J8 (Autodesk Fusion 360 design; units mm, degrees)
part number: 2026-05-31-14-41-56-693
Autodesk Fusion 360 part; units mm, degrees
sketch "Sketch1" plane through (0, 0, 0) normal (0, 0, 1) x (1, 0, 0)
  circle A0 centre (0, 0) radius 19.2
  dimension "d1" = 38.4
  constraint coincident A0.centre origin
  measures "d1" diameter of A0
extrude "Extrude1" add sketch "Sketch1" along normal blind 5
sketch "Sketch2" plane through (0, 0, 0) normal (0, 0, 1) x (1, 0, 0)
sketch "Sketch3" plane through (0, 0, 5) normal (0, 0, 1) x (-1, 0, 0)
  circle A0 centre (0, 0) radius 19.2
  circle A1 centre (0, 0) radius 15.2
  dimension "d4" = -4
extrude "Extrude2" add sketch "Sketch3" along normal blind 50
sketch "Sketch4" plane through (0, 0, 0) normal (0, 0, -1) x (1, 0, 0)
  circle A0 centre (0, 0) radius 19.2
  line L0 (-2, -22) -> (4, -22)
  line L1 (4, -22) -> (4, 22)
  line L2 (4, 22) -> (-4, 22)
  line L3 (-4, 22) -> (-4, -22)
  line L4 (-4, -22) -> (-2, -22)
  constraint horizontal L0
  constraint perpendicular L0 L1
  constraint perpendicular L1 L2
  constraint perpendicular L2 L3
  constraint perpendicular L3 L4
extrude "Extrude3" add sketch "Sketch4" along normal blind 5 contours A0 L1 L3 | A0 L1 L2 L3 | A0 L0 L1 L3 L4
extrude "Extrude4" add 2 faces at (0.4474, 21.051, 0) (0.4474, -21.051, 0) along direction (0, 0, 1) blind 5
sketch "Sketch5" plane through (0, 0, -5) normal (0, 0, -1) x (1, 0, 0)
  line L0 (-4, -22) -> (4, -22)
  line L1 (4, -22) -> (4, 22)
  line L2 (4, 22) -> (-4, 22)
  line L3 (-4, 22) -> (-4, -22)
  line L4 (4, -19) -> (-4, -19)
  line L5 (-4, -19) -> (-4, -22)
  line L6 (-4, -22) -> (4, -22)
  line L7 (4, -22) -> (4, -19)
  line L8 (-4, 22) -> (4, 22)
  line L9 (4, 22) -> (4, 19)
  line L10 (4, 19) -> (-4, 19)
  line L11 (-4, 19) -> (-4, 22)
  constraint horizontal L4
  constraint vertical L5
  constraint horizontal L6
  constraint vertical L7
  constraint coincident L0.start L3.end
  constraint coincident L1 L4.start
  constraint horizontal L8
  constraint vertical L9
  constraint horizontal L10
  constraint vertical L11
  constraint coincident L2.end L3.start
extrude "Extrude5" add sketch "Sketch5" along normal blind 20 contours L0 L1 L3 L4 L5 L6 L7 | L1 L2 L3 L8 L9 L10 L11
extrude "Extrude6" add 2 faces at (-1.3333, 20, -25) (-1.3333, -21, -25) along direction (0, 0, -1) blind 10
sketch "Sketch6" plane through (0, -19, 0) normal (0, 1, 0) x (-1, 0, 0)
  line L0 (4, -5) -> (-4, -5)
  line L1 (-4, -5) -> (-4, -35)
  line L2 (-4, -35) -> (4, -35)
  line L3 (4, -35) -> (4, -5)
  line L4 (0, -5) -> (0, -28)
  circle A0 centre (0, -28) radius 4
  dimension "d16" = 23
  dimension "d17" = 8
  constraint midpoint L0 L4.start
  constraint perpendicular L0 L4
  constraint coincident L4.end A0.centre
  measures "d16" distance of L4.start L4.end
  measures "d17" diameter of A0
extrude "Extrude7" add 1 faces at (-4, 6.2596, -3.3333) along direction (-1, 0, 0) blind 2
extrude "Extrude8" add 1 faces at (4, -6.2596, -3.3333) along direction (1, 0, 0) blind 2
extrude "Extrude9" cut sketch "Sketch6" along normal blind 49 contours A0
sketch "Sketch7" plane through (0, -19, 0) normal (0, 1, 0) x (-1, 0, 0)
  line L0 (6, -5) -> (-6, -5)
  line L1 (-6, -5) -> (-6, -35)
  line L2 (-6, -35) -> (6, -35)
  line L3 (6, -35) -> (6, -5)
  circle A0 centre (0, -28) radius 4.0311
extrude "Extrude10" cut sketch "Sketch7" against normal blind 12 contours A0
fillet "Fillet1" radius 4 1 edges at (6, 0, -5)
fillet "Fillet2" radius 4 1 edges at (-6, 0, -5)
fillet "Fillet3" radius 3 1 edges at (0, 22, 5)
fillet "Fillet4" radius 3 1 edges at (0, -22, 5)
fillet "Fillet5" radius 6 2 edges at (6, -20.5, -35) (6, 20.5, -35)
fillet "Fillet6" radius 6 2 edges at (-6, 20.5, -35) (-6, -20.5, -35)
